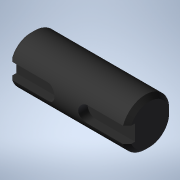
# Autodesk Inventor part: SSFHKR6-15-KA0-A6-KB9-B6_s
Saved by Autodesk Inventor 2021 (Build 250183000, 183)
## iProperties
Created: 2025-02-08
Part Number: SSFHKR6-15-KA0-A6-KB9-B6_s
Material: Generic
Catalog Web Link: www.cadenas.de
Description: NSFMKR, SFMKR, PSFMKR, SSFMKR, NSFHKR, SFHKR, PSFHKR, SSFHKR, NSFGKR, SFGKR, PSFGKR, SSFGKR, AHFGKR_shafts-Rotary Shafts - Straight with Keyway -
Vendor: MISUMI
Document SubType Name: Modeling
Designer: psAdmin
Manufacturer: MISUMI
Mass: 0.393669 g
Surface Area: 3.50809 cm^2
Volume: 0.393669 cm^3
Density: 1 g/cm^3
Appearance: PSOLRGB-175-175-175
Category: PARTsolutions
Company: MISUMI
Title: SSFHKR6-15-KA0-A6-KB9-B6
Author: Cadenas PARTsolutions
Comments: Rotary Shafts - Straight with Keyway -
PSOL_IDENT_0: {$CADENAS_DATA/23d-libs/misumi/metric/11_rotary_shafts/11_components/psfgkr/psfgkr.prj},499 {VTYP=3D
PSOL_IDENT_1: },{NB=SSFHKR6-15-KA0-A6-KB9-B6_s},{LINA=SSFHKR6-15-KA0-A6-KB9-B6},{NN=NSFMKR, SFMKR, PSFMKR, SSFMKR,
PSOL_IDENT_2: NSFHKR, SFHKR, PSFHKR, SSFHKR, NSFGKR, SFGKR, PSFGKR, SSFGKR, AHFGKR_shafts},{DATE=17.01.2024 00:02
PSOL_IDENT_3: :17},{GEOMDATE=27.12.2023 10:05:23},{VERSION=},{LINEID=10},{WBVAR=TS,MAT,ST,ALT1,L,NOK,KA,A,KB,B,KC,
PSOL_IDENT_4: C,ALT3,FC,GALT3,WFC,J,WALT3,V,ALT4,SFC,SGALT4,AG,ALT10,KWC,ALT11,WC,ALT6,TA,TB,ALT5,UC,ALT7,SC,ALT32
PSOL_IDENT_5: ,CD},{WBNUMERIC=L,KA,A,KB,B,KC,C,FC,GALT3,WFC,J,WALT3,V,SFC,SGALT4,AG,KWC,WC,TA,TB,UC,SC}  {NB=SSFHK
PSOL_IDENT_6: R6-15-KA0-A6-KB9-B6_s},{LINA=SSFHKR6-15-KA0-A6-KB9-B6},{KT=DUMMY},{PN=SSFHKR6-15-KA0-A6-KB9-B6},{TYP
PSOL_IDENT_7: E=SSFHKR},{TS=H},{TSALG= 'M','h9 (Cold-drawn)','H','h7 (Ground)','G','g6 (Ground)' },{MAT=SUS304},{M
PSOL_IDENT_8: ATALG= 'S45C','S45C Equivalent','SUS304','304 Stainless Steel' },{ST=-},{STALG= '-','-' },{D=6},{ALT
PSOL_IDENT_9: 1=},{L=15.0},{LALG=[15:500/0.1]},{LMIN=15},{LMAX=500},{NOK=2},{NOKALG= '1', 'with 1 Key Groove', '2'
PSOL_IDENT_10: , 'with 2 Key Grooves', '3'  , 'with 3 Key Grooves'},{BB=2},{TT=1.2},{KA=0.0},{KAALG=[0:9/0.1]},{K
PSOL_IDENT_11: AMIN=0},{KAMAX1=13},{KAMAX2=9},{KAMAX3=5},{A=6.0},{AALG=[2:11/0.1]},{AMIN=2},{AMAX1=15},{AMAX2=11},{
PSOL_IDENT_12: AMAX3=7},{KAPN=-KA0-A6},{KB=9.0},{KBALG=[8:13/0.1]},{KBMIN=8},{KBMAX1=13},{KBMAX2=9},{B=6.0},{BALG=[
PSOL_IDENT_13: 2:6/0.1]},{BMIN=2},{BMAX1=6},{BMAX2=2},{KBPN=-KB9-B6},{KC=0.0},{KCALG=[0]},{KCMIN=17},{KCMAX=13},{C=
PSOL_IDENT_14: 0.0},{CALG=[0]},{CMIN=2},{CMAX=15},{KCPN=},{CIFKA=1},{CIFKB=1},{CIFKC=3},{ALT3=},{ALT3ALG= '', 'w/o
PSOL_IDENT_15: Set Screw Flat','FC','with FC (Adds a Set Screw Flat)','WFC','with WFC (Adds Two Set Screw Flats)','
PSOL_IDENT_16: FCWFC','with FC + WFC (Adds Three Set Screw Flats)' },{ALT3PN=},{FC=0},{FCALG=[0]},{FCMIN=0},{FCMAX=
PSOL_IDENT_17: 14},{GALT3=0},{GALT3ALG=[0]},{GALT3MIN=1},{GALT3MAX=15},{GALT3MAX2=9},{GALT3MAX3=12},{WFC=0},{WFCALG=
PSOL_IDENT_18: [0]},{WFCMIN=0},{WFCMIN2=2},{WFCMAX=11},{WFCMAX2=-3},{WFCMAX3=-4},{J=0},{JALG=[0]},{JMIN=1},{JMAX=12
PSOL_IDENT_19: },{JMAX2=-2},{JMAX3=-5},{WALT3=0},{WALT3ALG=[0]},{WALT3MIN=0},{WALT3MIN2=17},{WALT3MAX=12},{WALT3MAX
PSOL_IDENT_20: 2=12},{V=0},{VALG=[0]},{VMIN=1},{VMAX=13},{VMAX3=13},{CIFFC=0},{ALT4=},{ALT4ALG= '', 'w/o SFC (2 Set
PSOL_IDENT_21: Screw Flats (Angle Specified))', 'SFC' , 'with SFC (2 Set Screw Flats (Angle Specified))'},{ALT4PN=
PSOL_IDENT_22: },{SFC=0},{SFCALG=[0]},{SFCMIN=0},{SFCMAX=14},{SGALT4=0},{SGALT4ALG=[0]},{SGALT4MIN=1},{SGALT4MAX=15
PSOL_IDENT_23: },{AG=0},{AGALG=[0]},{H=0},{CIFSFC=0},{ALT10=},{ALT10ALG= '','Not applicable' },{ALT10PN=},{KWC=0},{
PSOL_IDENT_24: KWCALG=[0]},{KWCMIN=1},{KWCMAX=6.5},{WALT10=0},{ALT11=},{ALT11ALG= '','Not applicable' },{ALT11PN=},
PSOL_IDENT_25: {WC=0.0},{WCALG=[0]},{ALT6=},{ALT6ALG= '','w/o Retaining Ring Groove','TA','with TA (Retaining Ring
PSOL_IDENT_26: Groove)','TB','with TB (Retaining Ring Groove)','TATB','with TA + TB (Two Retaining Ring Grooves)' }
PSOL_IDENT_27: ,{ALT6PN=},{TA=0.0},{TAALG=[0]},{TAMIN=2},{TAMAX=0},{TB=0.0},{TBALG=[0]},{TBMIN=2},{TBMAX=0},{DDALT6=
PSOL_IDENT_28: 0.0},{MM=0.00},{ALT5=},{ALT5ALG= '', 'w/o UC (Slit Cam Groove)', 'UC', 'with UC (Slit Cam Groove)'},
PSOL_IDENT_29: {ALT5PN=},{UC=0},{UCALG=[0]},{UCMIN=1},{UCMAX=10},{DD=0},{LL1=0},{ALT7=},{ALT7ALG= '', 'w/o SC (Wren
PSOL_IDENT_30: ch Flats)', 'SC', 'with SC (Wrench Flats)'},{ALT7PN=},{SC=0},{SCALG=[0]},{SCMIN=0},{SCMAX=7},{WALT7=
PSOL_IDENT_31: 0},{LL2=0},{LL2ALG=8},{CIFSC=0},{ALT32=},{ALT32ALG=  '','w/o CD (Changes Part D Chamfering)','CD', '
PSOL_IDENT_32: with CD (Changes Part D Chamfering)' },{ALT32PN=},{CD=},{CDALG= '','N/A' },{CD3D=0.5},{CIF32=0},{CIF
PSOL_IDENT_33: 320=0},{CIF32FC=0},{CIF32WFC=0},{CIF32WALT3=0},{ERRORPN=},{ERRORKGALT3=OK},{ERRORKGALT4=OK},{ERRORKG
PSOL_IDENT_34: ALT5=OK},{ERRORKGALT7=OK},{ERRORKGALT10=OK},{ERRORALT34=OK},{ERRORALT35=OK},{ERRORALT37=OK},{ERRORAL
PSOL_IDENT_35: T310=OK},{ERRORALT45=OK},{ERRORALT47=OK},{ERRORALT410=OK},{ERRORALT57=OK},{ERRORALT510=OK},{ERRORALT
PSOL_IDENT_36: 710=OK},{ERRORALT36=OK},{ERRORALT46=OK},{ERRORALT56=OK},{ERRORALT67=OK},{ERRORALT610=OK},{ERRORKGALT
PSOL_IDENT_37: 6=OK},{CIFTA=0},{CIFTB=0}
NB: SSFHKR6-15-KA0-A6-KB9-B6_s
NN: NSFMKR, SFMKR, PSFMKR, SSFMKR, NSFHKR, SFHKR, PSFHKR, SSFHKR, NSFGKR, SFGKR, PSFGKR, SSFGKR, AHFGKR_shafts
NT: Rotary Shafts - Straight with Keyway -
NBSYN: $PN._s
LINA: SSFHKR6-15-KA0-A6-KB9-B6
CATALOG: Misumi
PN: SSFHKR6-15-KA0-A6-KB9-B6
TYPE: SSFHKR
TS: h7 (Ground)
MAT: 304 Stainless Steel
ST: -
D: 6
ALT1: w/o LKC (Changes L Tolerance)
L: 15
NOK: with 2 Key Grooves
KA: 0
A: 6
KB: 9
B: 6
KC: 0
C: 0
ALT3: w/o Set Screw Flat
FC: 0
GALT3: 0
WFC: 0
J: 0
WALT3: 0
V: 0
ALT4: w/o SFC (2 Set Screw Flats (Angle Specified))
SFC: 0
SGALT4: 0
AG: 0
H: 0
ALT10: Not applicable
KWC: 0
ALT11: Not applicable
WC: 0
ALT6: w/o Retaining Ring Groove
TA: 0
TB: 0
DDALT6: 0
MM: 0
ALT5: w/o UC (Slit Cam Groove)
UC: 0
LL1: 0
ALT7: w/o SC (Wrench Flats)
SC: 0
WALT7: 0
LL2: 0
ALT32: w/o CD (Changes Part D Chamfering)
CD: N/A
SUPPLIER: MISUMI
ARTICLENO: SSFHKR6-15-KA0-A6-KB9-B6_s
BOMINFO: SSFHKR6-15-KA0-A6-KB9-B6
CREATOR: CADENAS GmbH
Autodesk Inventor part; units mm, degrees
ref_plane "YZ Plane" through (0, 0, 0) normal (1, 0, 0) x (0, 1, 0)
ref_plane "XZ Plane" through (0, 0, 0) normal (0, 1, 0) x (-1, 0, 0)
ref_plane "XY Plane" through (0, 0, 0) normal (0, 0, 1) x (1, 0, 0)
sketch "Sketch_1" plane through (0, 0, 0) normal (0, 1, 0) x (-1, 0, 0)
  line L0 (-15, 0) -> (0, 0)
  line L1 (0, 0) -> (0, -2.5)
  line L2 (0, -2.5) -> (-0.5, -3)
  line L3 (-0.5, -3) -> (-14.5, -3)
  line L4 (-14.5, -3) -> (-15, -2.5)
  line L5 (-15, -2.5) -> (-15, 0)
  line L6 (-15, 0) -> (0, 0)
  constraints: 14 end point
revolve "Revolution1" add sketch "Sketch_1" angle 360 about axis through (15, 0, 0) along (1, 0, 0)
sketch "_____9" plane through (0, 0, 3) normal (0, 0, 1) x (1, 0, 0)
  line L0 (0, 1) -> (0, -1)
  line L1 (0, -1) -> (5, -1)
  arc A0 (5, -1) -> (5, 1) centre (5, 0) ccw
  line L2 (5, 1) -> (0, 1)
  constraints: 6 end point, 2 point on circle, 1 centre point
extrude "Extrusion1" cut sketch "_____9" against normal blind 1.2
sketch "_____14" plane through (0, 0, 3) normal (0, 0, 1) x (1, 0, 0)
  arc A0 (10, 1) -> (10, -1) centre (10, 0) ccw
  line L0 (10, -1) -> (15, -1)
  line L1 (15, -1) -> (15, 1)
  line L2 (15, 1) -> (10, 1)
  constraints: 6 end point, 2 point on circle, 1 centre point
extrude "Extrusion2" cut sketch "_____14" against normal blind 1.2
body "Solid1"
